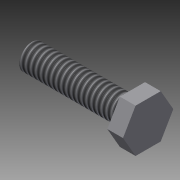
# Autodesk Inventor part: bolt
Saved by Autodesk Inventor 2015 (Build 190159000, 159)
## iProperties
Created: 2015-02-22
Part Number: bolt
Material: Generic
Document SubType Name: Modeling
Designer: Jarod
Density: 1 g/cm^3
Appearance: Default
Author: Jarod
Autodesk Inventor part; units mm, degrees
ref_plane "YZ Plane" through (0, 0, 0) normal (1, 0, 0) x (0, 1, 0)
ref_plane "XZ Plane" through (0, 0, 0) normal (0, 1, 0) x (-1, 0, 0)
ref_plane "XY Plane" through (0, 0, 0) normal (0, 0, 1) x (1, 0, 0)
sketch "Sketch1" plane through (0, 0, 0) normal (1, 0, 0) x (0, 1, 0)
  circle A0 centre (0, 0) radius 3.175
  dimension "d0" = 6.35
  constraints: 1 centre point, 1 coincident
  measures "d0" diameter of A0
extrude "Extrusion1" add sketch "Sketch1" along normal blind 25.4
thread "Thread1" size "1/4-20 UNC" class "2A" standard "ANSI Unified Screw Threads" full length
sketch "Sketch2" plane through (25.4, 0, 0) normal (1, 0, 0) x (0, 0, -1)
  circle A0 centre (0, 0) radius 6.35
  line L0 (6.35, 0) -> (3.175, -5.4993)
  line L1 (3.175, -5.4993) -> (-3.175, -5.4993)
  line L2 (-3.175, -5.4993) -> (-6.35, 0)
  line L3 (-6.35, 0) -> (-3.175, 5.4993)
  line L4 (-3.175, 5.4993) -> (3.175, 5.4993)
  line L5 (3.175, 5.4993) -> (6.35, 0)
  dimension "d5" = 12.7
  constraints: 12 end point, 2 coincident, 1 horizontal alignment, 15 other
extrude "Extrusion2" add sketch "Sketch2" along normal blind 3.9688 contours L0 L1 L2 L3 L4 L5
body "Solid1"
